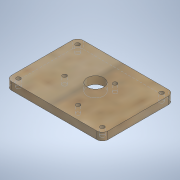
# Autodesk Inventor part: 上下直動t5.5
Saved by Autodesk Inventor 2020.3 (Build 243373000, 373)
## iProperties
Created: 2020-07-05
Part Number: 上下直動t5.5
Material: 木材 (カエデ材)
Document SubType Name: Modeling
Designer: totot
Density: 0.67 g/cm^3
Appearance: ナチュラル カエデ材 - 光沢 濃い着色
Author: totot
Autodesk Inventor part; units mm, degrees
ref_plane "YZ Plane" through (0, 0, 0) normal (1, 0, 0) x (0, 1, 0)
ref_plane "XZ Plane" through (0, 0, 0) normal (0, 1, 0) x (-1, 0, 0)
ref_plane "XY Plane" through (0, 0, 0) normal (0, 0, 1) x (1, 0, 0)
sketch "スケッチ1" plane through (0, 0, 0) normal (0, 1, 0) x (-1, 0, 0)
  line L0 (0, 0) -> (-70, 0)
  line L1 (-70, 0) -> (-70, 57)
  line L2 (-70, 57) -> (0, 57)
  line L3 (0, 57) -> (0, 0)
  dimension "d2" = 70
  dimension "d3" = 57
  constraints: 8 end point, 2 parallel, 1 horizontal, 1 perpendicular
  measures "d2" distance of L0.start L0.end
  measures "d3" distance between parallel lines of L2 L0
extrude "押し出し1" add sketch "スケッチ1" along normal blind 5.5
sketch "スケッチ2" plane through (0, 0, 0) normal (0, -1, 0) x (1, 0, 0)
  line L0 (70, 0) -> (0, 0) projected
  line L1 (70, 57) -> (70, 0) projected
  line L2 (0, 0) -> (0, 57) projected
  line L3 (0, 57) -> (70, 57) projected
  point P0 (65.5, 4.5)
  point P1 (4.5, 4.5)
  point P2 (4.5, 52.5)
  point P3 (65.5, 52.5)
  dimension "d4" = 4.5
  dimension "d5" = 4.5
  dimension "d6" = 4.5
  dimension "d7" = 4.5
  dimension "d8" = 4.5
  dimension "d9" = 4.5
  dimension "d10" = 4.5
  dimension "d11" = 4.5
  measures "d4" distance from line of point (65.5, 4.5) L0
  measures "d5" distance from line of L1 point (65.5, 4.5)
  measures "d6" distance from line of L0 point (4.5, 4.5)
  measures "d7" distance from line of L2 point (4.5, 4.5)
  measures "d8" distance from line of L3 point (65.5, 52.5)
  measures "d9" distance from line of L1 point (65.5, 52.5)
  measures "d10" distance from line of L2 point (4.5, 52.5)
  measures "d11" distance from line of L3 point (4.5, 52.5)
hole "穴1" at (65.5, 0, 4.5) at (4.5, 0, 4.5) at (4.5, 0, 52.5) at (65.5, 0, 52.5) direction (0, 1, 0) diameter 3 end through all
fillet "フィレット1" radius 4 4 edges at (70, 2.75, 0) (0, 2.75, 0) (70, 2.75, 57) (0, 2.75, 57)
sketch "スケッチ3" plane through (0, 0, 0) normal (0, -1, 0) x (1, 0, 0)
  circle A0 centre (28, 29) radius 15.5
  line L0 (0, 4) -> (0, 53) projected
  line L1 (70, 53) -> (70, 4) projected
  line L2 (4, 57) -> (66, 57) projected
  line L3 (28, 29) -> (12.5, 29)
  line L4 (28, 29) -> (35.75, 15.5766)
  line L5 (28, 29) -> (35.75, 42.4234)
  point P0 (0, 0)
  dimension "d20" = 31
  dimension "d21" = 70
  dimension "d22" = 42
  dimension "d23" = 28
  dimension "d24" = 120
  dimension "d25" = 120
  constraints: 6 end point, 3 coincident, 3 point on circle, 1 centre point, 1 horizontal
  measures "d20" diameter of A0
  measures "d21" distance between parallel lines of L0 L1
  measures "d22" distance from line of L1 L3.start
  measures "d23" distance from line of L2 L3.start
  measures "d24" angle of L5 L4
  measures "d25" angle of L3 L5
hole "穴2" at (35.75, 0, 15.5766) at (35.75, 0, 42.4234) at (12.5, 0, 29) direction (0, 1, 0) diameter 3 end through all
sketch "スケッチ4" plane through (0, 0, 0) normal (0, -1, 0) x (1, 0, 0)
  circle A0 centre (28, 22) radius 6
  line L0 (70, 53) -> (70, 4) projected
  line L1 (4, 57) -> (66, 57) projected
  point P0 (0, 0)
  dimension "d33" = 12
  dimension "d34" = 42
  dimension "d35" = 35
  constraints: 1 centre point
  measures "d33" diameter of A0
  measures "d34" distance from line of A0.centre L0
  measures "d35" distance from line of A0.centre L1
extrude "押し出し2" cut sketch "スケッチ4" against normal through all
equation "\"d7\" = d5"
equation "\"d8\" = d5"
equation "\"d9\" = d5"
equation "\"d10\" = d5"
equation "\"d11\" = d5"
